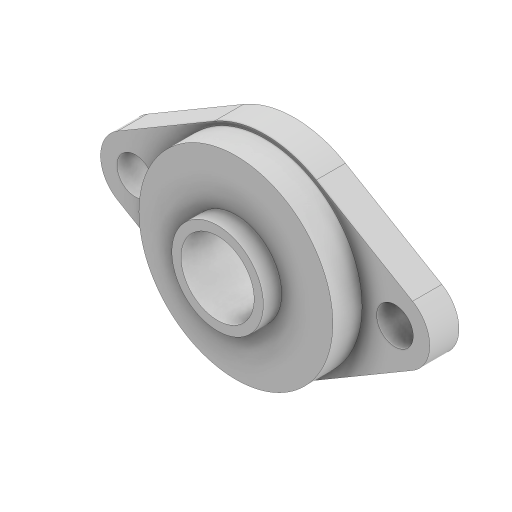
# Autodesk Inventor part: RODAMIENTO DE PARED
Saved by Autodesk Inventor 2024 (Build 280153000, 153)
## iProperties
Created: 2024-06-28
Part Number: RODAMIENTO DE PARED
Material: Generic
Document SubType Name: Modeling
Designer: Jhuliams
Density: 1 g/cm^3
Appearance: Default
Author: Jhuliams
Autodesk Inventor part; units mm, degrees
ref_plane "YZ Plane" through (0, 0, 0) normal (1, 0, 0) x (0, 1, 0)
ref_plane "XZ Plane" through (0, 0, 0) normal (0, 1, 0) x (-1, 0, 0)
ref_plane "XY Plane" through (0, 0, 0) normal (0, 0, 1) x (1, 0, 0)
sketch "Sketch1" plane through (0, 0, 0) normal (0, 0, 1) x (1, 0, 0)
  line L0 (-26, 0) -> (-35.5, 0)
  circle A0 centre (-35.5, 0) radius 5
  line L1 (0, 0) -> (0, 5.7402)
  arc A1 (-40.3169, 8.1883) -> (-40.3169, -8.1883) centre (-35.5, 0) ccw
  line L2 (-40.3169, 8.1883) -> (-13.9437, 23.7028)
  line L3 (-40.3169, -8.1883) -> (-13.9437, -23.7028)
  arc A2 (-13.9437, -23.7028) -> (0, -27.5) centre (0, 0) ccw
  arc A3 (0, 27.5) -> (-13.9437, 23.7028) centre (0, 0) ccw
  line L4 (26, 0) -> (35.5, 0)
  circle A4 centre (35.5, 0) radius 5
  arc A5 (40.3169, -8.1883) -> (40.3169, 8.1883) centre (35.5, 0) ccw
  line L5 (40.3169, 8.1883) -> (13.9437, 23.7028)
  line L6 (40.3169, -8.1883) -> (13.9437, -23.7028)
  arc A6 (0, -27.5) -> (13.9437, -23.7028) centre (0, 0) ccw
  arc A7 (13.9437, 23.7028) -> (0, 27.5) centre (0, 0) ccw
  dimension "d1" = 35.5
  dimension "d2" = 10
  dimension "d15" = 19
  constraints: 14 end point, 12 point on circle, 10 symmetric about line, 8 centre point, 6 coincident, 2 point on line, 2 tangent, 1 horizontal, 1 vertical, 4 other
  measures "d1" distance of L1.start L0.end
  measures "d2" diameter of A0
  measures "d15" diameter of A1
extrude "Extrusion1" add sketch "Sketch1" along normal blind 8
sketch "Sketch2" plane through (0, 0, 8) normal (0, 0, 1) x (1, 0, 0)
  circle A0 centre (0, 0) radius 26.5
  dimension "d6" = 53
  constraints: 1 centre point, 1 coincident
  measures "d6" diameter of A0
extrude "Extrusion2" add sketch "Sketch2" along normal blind 8
sketch "Sketch3" plane through (0, 0, 16) normal (0, 0, 1) x (1, 0, 0)
  circle A0 centre (0, 0) radius 10
  circle A1 centre (0, 0) radius 12.5
  dimension "d9" = 20
  dimension "d10" = 25
  constraints: 2 centre point, 2 coincident
  measures "d9" diameter of A0
  measures "d10" diameter of A1
extrude "Extrusion3" add sketch "Sketch3" along normal blind 5
sketch "Sketch4" plane through (0, 0, 16) normal (0, 0, 1) x (1, 0, 0)
  circle A0 centre (0, 0) radius 10 projected
extrude "Extrusion4" cut sketch "Sketch4" against normal blind 30
body "Solid1"
